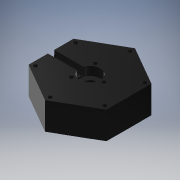
# Autodesk Inventor part: Spur Gear2
Saved by Autodesk Inventor 2017 (Build 210142000, 142)
## iProperties
Created: 2018-10-09
Part Number: Spur Gear2
Material: ABS Plastic
Document SubType Name: Modeling
Designer: Zach
Categories: <?xml version="1.0" encoding="UTF-16"?> <MemberInstance><Categories><FamilyTemplate><FamilyTemplateParameter ValueType="xs:double" Id="1" ObjectReferenceKey="da_z" ObjectType="kUserParameterObject"/><FamilyTemplateParameter ValueType="xs:double" Id="2" ObjectReferenceKey="da_b" ObjectType="kUserParameterObject"/><FamilyTemplateParameter ValueType="xs:double" Id="3" ObjectReferenceKey="da_beta" ObjectType="kUserParameterObject"/><FamilyTemplateParameter ValueType="xs:double" Id="4" ObjectReferenceKey="da_da" ObjectType="kUserParameterObject"/><FamilyTemplateParameter ValueType="xs:double" Id="5" ObjectReferenceKey="da_aw" ObjectType="kUserParameterObject"/><FamilyTemplateParameter ValueType="xs:string" Id="6" ObjectReferenceKey="EAIAABAAAACIAQAAAAAAAIAAAAAAAAAA" ObjectType="83910656" SubObjectId="SurfaceGeometry"/></FamilyTemplate><ParamToTemplateMap><ParamToTemplate CategoryParameter="//CategoryParameter[@InternalName='046C89C9-8512-4d59-83FE-43B91F4F132A']" TemplateParameter="1"/><ParamToTemplate CategoryParameter="//CategoryParameter[@InternalName='2552DF32-E462-4b46-AEBF-C6C7768E72AC']" TemplateParameter="2"/><ParamToTemplate CategoryParameter="//CategoryParameter[@InternalName='C9EE641D-15FC-4fae-A226-E94C4372FDD7']" TemplateParameter="3"/><ParamToTemplate><ParamToTemplate CategoryParameter="//CategoryParameter[@InternalName='00B6519A-459B-49c7-AD84-2E56D39A5744']" ConstantValue="0.000000"/></ParamToTemplate><ParamToTemplate><ParamToTemplate CategoryParameter="//CategoryParameter[@InternalName='04B31F0E-C7A6-4894-AA32-9629BEFACF47']" ConstantValue="1.000000"/></ParamToTemplate><ParamToTemplate><ParamToTemplate CategoryParameter="//CategoryParameter[@InternalName='43CBEC2E-7847-49e7-A936-2F7889FCB2D9']" ConstantValue="0.250000"/></ParamToTemplate><ParamToTemplate><ParamToTemplate CategoryParameter="//CategoryParameter[@InternalName='B1EFC894-105D-4ebd-86BF-FA20ED196853']" ConstantValue="0.350000"/></ParamToTemplate><ParamToTemplate><ParamToTemplate CategoryParameter="//CategoryParameter[@InternalName='51175063-3D10-4879-93E8-6246FE8B403D']" ConstantValue="2060000000.000000"/></ParamToTemplate><ParamToTemplate><ParamToTemplate CategoryParameter="//CategoryParameter[@InternalName='A3A52E27-4454-46a9-B0BD-C932399B70AF']" ConstantValue="0.300000"/></ParamToTemplate><ParamToTemplate><ParamToTemplate CategoryParameter="//CategoryParameter[@InternalName='91B76062-C214-41d9-B1B9-14D2AB99603D']" ConstantValue="0.200000"/></ParamToTemplate><ParamToTemplate><ParamToTemplate CategoryParameter="//CategoryParameter[@InternalName='374E806E-8B8A-4dda-A9AA-1039D6500AD2']" ConstantValue="5.000000"/></ParamToTemplate><ParamToTemplate><ParamToTemplate CategoryParameter="//CategoryParameter[@InternalName='2D373A89-B862-43d6-8D0B-0CBF12AB9F6C']" ConstantValue="0.392699"/></ParamToTemplate><ParamToTemplate CategoryParameter="//CategoryParameter[@InternalName='37777632-D6A2-4fac-9D53-DB8ACD95C989']" TemplateParameter="4"/><ParamToTemplate CategoryParameter="//CategoryParameter[@InternalName='FD1017F1-B727-4f7e-9707-0F86F1FF9423']" TemplateParameter="5"/><ParamToTemplate><ParamToTemplate CategoryParameter="//CategoryParameter[@InternalName='9E1B4470-B2D3-4ff1-B813-535BB4CDF51A']" ConstantValue="3520000.000000"/></ParamToTemplate><ParamToTemplate><ParamToTemplate CategoryParameter="//CategoryParameter[@InternalName='F8452263-BFF6-458c-9FB1-07C4B99E95CD']" ConstantValue="11400000.000000"/></ParamToTemplate><ParamToTemplate><ParamToTemplate CategoryParameter="//CategoryParameter[@InternalName='3E3BB259-FD49-497f-8171-6EBC954A3479']" ConstantValue="2.000000"/></ParamToTemplate><ParamToTemplate CategoryParameter="//CategoryParameter[@InternalName='27C3BAF2-7550-4e4b-AE2C-0DB134B7D9B7']" TemplateParameter="6"/></ParamToTemplateMap><Category DisplayName="Gear" InternalName="DC85795E-93AB-48d5-8EEE-5A27447B64BD" Mnemonic="Gear"><CategoryParameter DisplayName="z" InternalName="046C89C9-8512-4d59-83FE-43B91F4F132A" Mnemonic="z"/><CategoryParameter DisplayName="b" InternalName="2552DF32-E462-4b46-AEBF-C6C7768E72AC" Mnemonic="b"/><CategoryParameter DisplayName="||b|" InternalName="C9EE641D-15FC-4fae-A226-E94C4372FDD7" Mnemonic="beta"/><CategoryParameter DisplayName="x" InternalName="00B6519A-459B-49c7-AD84-2E56D39A5744" Mnemonic="x"/><CategoryParameter DisplayName="a*" InternalName="04B31F0E-C7A6-4894-AA32-9629BEFACF47" Mnemonic="a"/><CategoryParameter DisplayName="c*" InternalName="43CBEC2E-7847-49e7-A936-2F7889FCB2D9" Mnemonic="c"/><CategoryParameter DisplayName="r|.f|*" InternalName="B1EFC894-105D-4ebd-86BF-FA20ED196853" Mnemonic="rf"/><CategoryParameter DisplayName="E" InternalName="51175063-3D10-4879-93E8-6246FE8B403D" Mnemonic="E"/><CategoryParameter DisplayName="||m|" InternalName="A3A52E27-4454-46a9-B0BD-C932399B70AF" Mnemonic="mi"/><Category DisplayName="SpurGear" InternalName="26C5A22E-A91E-4dfd-A3B3-23CCAFAE1764" Mnemonic="SpurGear"><CategoryParameter DisplayName="m" InternalName="91B76062-C214-41d9-B1B9-14D2AB99603D" Mnemonic="m"/><CategoryParameter DisplayName="P" InternalName="374E806E-8B8A-4dda-A9AA-1039D6500AD2" Mnemonic="PP"/><CategoryParameter DisplayName="||a|" InternalName="2D373A89-B862-43d6-8D0B-0CBF12AB9F6C" Mnemonic="alpha"/><CategoryParameter DisplayName="d|.a|" InternalName="37777632-D6A2-4fac-9D53-DB8ACD95C989" Mnemonic="da"/><CategoryParameter DisplayName="a|.w|" InternalName="FD1017F1-B727-4f7e-9707-0F86F1FF9423" Mnemonic="aw"/><CategoryParameter DisplayName="||s||.Flim|" InternalName="9E1B4470-B2D3-4ff1-B813-535BB4CDF51A" Mnemonic="sFlim"/><CategoryParameter DisplayName="||s||.Hlim|" InternalName="F8452263-BFF6-458c-9FB1-07C4B99E95CD" Mnemonic="sHlim"/><CategoryParameter DisplayName="type" InternalName="3E3BB259-FD49-497f-8171-6EBC954A3479" Mnemonic="type"/><Category DisplayName="InternalSpurGear" InternalName="7CF704F6-14A9-42f8-93CE-E71DF57C2B55" Mnemonic="InternalSpurGear"><CategoryParameter DisplayName="PitchDiameter" InternalName="27C3BAF2-7550-4e4b-AE2C-0DB134B7D9B7" Mnemonic="IDS_PITCHDIAM"/></Category></Category></Category></Categories></MemberInstance>
Density: 1.06 g/cm^3
Appearance: Smooth - Black
CustomPartVersion: 0
Author: Zach
Autodesk Inventor part; units mm, degrees
ref_plane "YZ Plane" through (0, 0, 0) normal (1, 0, 0) x (0, 1, 0)
ref_plane "XZ Plane" through (0, 0, 0) normal (0, 1, 0) x (-1, 0, 0)
ref_plane "XY Plane" through (0, 0, 0) normal (0, 0, 1) x (1, 0, 0)
sketch "Sketch1" plane through (0, 0, 0) normal (0, 0, 1) x (1, 0, 0)
  circle A0 centre (0, 0) radius 52.25
  dimension "d0" = 104.5
  constraints: 1 centre point
  measures "d0" diameter of A0
extrude "Extrusion1" add sketch "Sketch1" along normal blind 10
ref_plane "Work Plane2" through (0, 0, 5) normal (0, 0, 1) x (1, 0, 0)
sketch "Sketch2" plane through (0, 0, 0) normal (0, 0, -1) x (-1, 0, 0)
  circle A0 centre (0, 0) radius 52.25 projected
  circle A1 centre (0, 0) radius 45
  dimension "d3" = 90
  constraints: 1 centre point, 1 coincident
  measures "d3" diameter of A1
surface extrude "Pitch Diameter" sketch "Sketch2" against normal through all shown no curves A1
ref_plane "Work Plane8" through (0, 0, 0) normal (0.9975641, 0.0697565, 0) x (0, 0, 1)
ref_plane "Work Plane9" through (0, 0, 0) normal (1, 0, 0) x (0, 1, 0)
spur gear teeth "Spur Gear" teeth 45 pitch diameter 90 tip diameter 86.2612 root diameter 95 face width 10 start plane through (0, 0, 0) normal (0, 0, -1) x (-1, 0, 0)
sketch "Sketch3" plane through (0, 0, 10) normal (0, 0, 1) x (1, 0, 0)
  arc A0 (2.2573, -43.0715) -> (3.7591, -42.9665) centre (0, 0) ccw projected
  arc A1 (0.829, -47.4928) -> (2.2573, -43.0715) centre (-19.4558, -38.4984) ccw projected
  arc A2 (-0.829, -47.4928) -> (0.829, -47.4928) centre (0, 0) ccw projected
  arc A3 (-2.2573, -43.0715) -> (-0.829, -47.4928) centre (19.4558, -38.4984) ccw projected
  arc A4 (-3.7591, -42.9665) -> (-2.2573, -43.0715) centre (0, 0) ccw projected
  arc A5 (-5.7888, -47.1459) -> (-3.7591, -42.9665) centre (-24.6244, -35.4161) ccw projected
  arc A6 (-7.4306, -46.9152) -> (-5.7888, -47.1459) centre (0, 0) ccw projected
  arc A7 (-8.2297, -42.3382) -> (-7.4306, -46.9152) centre (13.9085, -40.8315) ccw projected
  arc A8 (-9.7023, -42.0252) -> (-8.2297, -42.3382) centre (0, 0) ccw projected
  arc A9 (-12.2939, -45.8815) -> (-9.7023, -42.0252) centre (-29.3137, -31.6443) ccw projected
  arc A10 (-13.8877, -45.4245) -> (-12.2939, -45.8815) centre (0, 0) ccw projected
  arc A11 (-14.0419, -40.7808) -> (-13.8877, -45.4245) centre (8.0905, -42.3698) ccw projected
  arc A12 (-15.4566, -40.2659) -> (-14.0419, -40.7808) centre (0, 0) ccw projected
  arc A13 (-18.5597, -43.724) -> (-15.4566, -40.2659) centre (-33.4325, -27.2567) ccw projected
  arc A14 (-20.0744, -43.0496) -> (-18.5597, -43.724) centre (0, 0) ccw projected
  arc A15 (-19.5809, -38.4296) -> (-20.0744, -43.0496) centre (2.115, -43.0835) ccw projected
  arc A16 (-20.9101, -37.7229) -> (-19.5809, -38.4296) centre (0, 0) ccw projected
  arc A17 (-24.4643, -40.7154) -> (-20.9101, -37.7229) centre (-36.9005, -22.3385) ccw projected
  arc A18 (-25.8704, -39.8369) -> (-24.4643, -40.7154) centre (0, 0) ccw projected
  arc A19 (-24.7387, -35.3305) -> (-25.8704, -39.8369) centre (-3.9016, -42.9585) ccw projected
  arc A20 (-25.9566, -34.4456) -> (-24.7387, -35.3305) centre (0, 0) ccw projected
  arc A21 (-29.8927, -36.9144) -> (-25.9566, -34.4456) centre (-39.6503, -16.9856) ccw projected
  arc A22 (-31.1628, -35.8487) -> (-29.8927, -36.9144) centre (0, 0) ccw projected
  arc A23 (-29.415, -31.5437) -> (-31.1628, -35.8487) centre (-9.8423, -41.9975) ccw projected
  arc A24 (-30.4979, -30.4979) -> (-29.415, -31.5437) centre (0, 0) ccw projected
  arc A25 (-34.7393, -32.3949) -> (-30.4979, -30.4979) centre (-41.6284, -11.302) ccw projected
  arc A26 (-35.8487, -31.1628) -> (-34.7393, -32.3949) centre (0, 0) ccw projected
  arc A27 (-33.5188, -27.143) -> (-35.8487, -31.1628) centre (-15.5915, -40.219) ccw projected
  arc A28 (-34.4456, -25.9566) -> (-33.5188, -27.143) centre (0, 0) ccw projected
  arc A29 (-38.9097, -27.2449) -> (-34.4456, -25.9566) centre (-42.7962, -5.3985) ccw projected
  arc A30 (-39.8369, -25.8704) -> (-38.9097, -27.2449) centre (0, 0) ccw projected
  arc A31 (-36.9701, -22.2139) -> (-39.8369, -25.8704) centre (-21.0371, -37.6576) ccw projected
  arc A32 (-37.7229, -20.9101) -> (-36.9701, -22.2139) centre (0, 0) ccw projected
  arc A33 (-42.3228, -21.5645) -> (-37.7229, -20.9101) centre (-43.131, 0.6101) ccw projected
  arc A34 (-43.0496, -20.0744) -> (-42.3228, -21.5645) centre (0, 0) ccw projected
  arc A35 (-39.7019, -16.8525) -> (-43.0496, -20.0744) centre (-26.0733, -34.3634) ccw projected
  arc A36 (-40.2659, -15.4566) -> (-39.7019, -16.8525) centre (0, 0) ccw projected
  arc A37 (-44.9121, -15.4645) -> (-40.2659, -15.4566) centre (-42.6264, 6.6069) ccw projected
  arc A38 (-45.4245, -13.8877) -> (-44.9121, -15.4645) centre (0, 0) ccw projected
  arc A39 (-41.6609, -11.163) -> (-45.4245, -13.8877) centre (-30.602, -30.4002) ccw projected
  arc A40 (-42.0252, -9.7023) -> (-41.6609, -11.163) centre (0, 0) ccw projected
  arc A41 (-46.6273, -9.0634) -> (-42.0252, -9.7023) centre (-41.292, 12.475) ccw projected
  arc A42 (-46.9152, -7.4306) -> (-46.6273, -9.0634) centre (0, 0) ccw projected
  arc A43 (-42.8091, -5.2563) -> (-46.9152, -7.4306) centre (-34.5351, -25.8454) ccw projected
  arc A44 (-42.9665, -3.7591) -> (-42.8091, -5.2563) centre (0, 0) ccw projected
  arc A45 (-47.4349, -2.486) -> (-42.9665, -3.7591) centre (-39.154, 18.1004) ccw projected
  arc A46 (-47.4928, -0.829) -> (-47.4349, -2.486) centre (0, 0) ccw projected
  arc A47 (-43.124, 0.7527) -> (-47.4928, -0.829) centre (-37.796, -20.7875) ccw projected
  arc A48 (-43.0715, 2.2573) -> (-43.124, 0.7527) centre (0, 0) ccw projected
  arc A49 (-47.3192, 4.1399) -> (-43.0715, 2.2573) centre (-36.2539, 23.3734) ccw projected
  arc A50 (-47.1459, 5.7888) -> (-47.3192, 4.1399) centre (0, 0) ccw projected
  arc A51 (-42.5996, 6.7471) -> (-47.1459, 5.7888) centre (-40.3212, -15.325) ccw projected
  arc A52 (-42.3382, 8.2297) -> (-42.5996, 6.7471) centre (0, 0) ccw projected
  arc A53 (-46.2826, 10.6852) -> (-42.3382, 8.2297) centre (-32.6481, 28.1915) ccw projected
  arc A54 (-45.8815, 12.2939) -> (-46.2826, 10.6852) centre (0, 0) ccw projected
  arc A55 (-41.246, 12.6102) -> (-45.8815, 12.2939) centre (-42.0617, -9.5642) ccw projected
  arc A56 (-40.7808, 14.0419) -> (-41.246, 12.6102) centre (0, 0) ccw projected
  arc A57 (-44.3451, 17.0225) -> (-40.7808, 14.0419) centre (-28.4069, 32.4609) ccw projected
  arc A58 (-43.724, 18.5597) -> (-44.3451, 17.0225) centre (0, 0) ccw projected
  arc A59 (-39.0896, 18.2278) -> (-43.724, 18.5597) centre (-42.9834, -3.6173) ccw projected
  arc A60 (-38.4296, 19.5809) -> (-39.0896, 18.2278) centre (0, 0) ccw projected
  arc A61 (-41.5444, 23.0285) -> (-38.4296, 19.5809) centre (-23.6127, 36.0984) ccw projected
  arc A62 (-40.7154, 24.4643) -> (-41.5444, 23.0285) centre (0, 0) ccw projected
  arc A63 (-36.1724, 23.4906) -> (-40.7154, 24.4643) centre (-43.0685, 2.4) ccw projected
  arc A64 (-35.3305, 24.7387) -> (-36.1724, 23.4906) centre (0, 0) ccw projected
  arc A65 (-37.9352, 28.5862) -> (-35.3305, 24.7387) centre (-18.359, 39.0334) ccw projected
  arc A66 (-36.9144, 29.8927) -> (-37.9352, 28.5862) centre (0, 0) ccw projected
  arc A67 (-32.5511, 28.2962) -> (-36.9144, 29.8927) centre (-42.3154, 8.3706) ccw projected
  arc A68 (-31.5437, 29.415) -> (-32.5511, 28.2962) centre (0, 0) ccw projected
  arc A69 (-33.5876, 33.5876) -> (-31.5437, 29.415) centre (-12.748, 41.2086) ccw projected
  arc A70 (-32.3949, 34.7393) -> (-33.5876, 33.5876) centre (0, 0) ccw projected
  arc A71 (-28.2962, 32.5511) -> (-32.3949, 34.7393) centre (-40.7386, 14.1783) ccw projected
  arc A72 (-27.143, 33.5188) -> (-28.2962, 32.5511) centre (0, 0) ccw projected
  arc A73 (-28.5862, 37.9352) -> (-27.143, 33.5188) centre (-6.8888, 42.5817) ccw projected
  arc A74 (-27.2449, 38.9097) -> (-28.5862, 37.9352) centre (0, 0) ccw projected
  arc A75 (-23.4906, 36.1724) -> (-27.2449, 38.9097) centre (-38.3689, 19.7101) ccw projected
  arc A76 (-22.2139, 36.9701) -> (-23.4906, 36.1724) centre (0, 0) ccw projected
  arc A77 (-23.0285, 41.5444) -> (-22.2139, 36.9701) centre (-0.8955, 43.126) ccw projected
  arc A78 (-21.5645, 42.3228) -> (-23.0285, 41.5444) centre (0, 0) ccw projected
  arc A79 (-18.2278, 39.0896) -> (-21.5645, 42.3228) centre (-35.2524, 24.8582) ccw projected
  arc A80 (-16.8525, 39.7019) -> (-18.2278, 39.0896) centre (0, 0) ccw projected
  arc A81 (-17.0225, 44.3451) -> (-16.8525, 39.7019) centre (5.1152, 42.831) ccw projected
  arc A82 (-15.4645, 44.9121) -> (-17.0225, 44.3451) centre (0, 0) ccw projected
  arc A83 (-12.6102, 41.246) -> (-15.4645, 44.9121) centre (-31.4497, 29.5224) ccw projected
  arc A84 (-11.163, 41.6609) -> (-12.6102, 41.246) centre (0, 0) ccw projected
  arc A85 (-10.6852, 46.2826) -> (-11.163, 41.6609) centre (11.0263, 41.7022) ccw projected
  arc A86 (-9.0634, 46.6273) -> (-10.6852, 46.2826) centre (0, 0) ccw projected
  arc A87 (-6.7471, 42.5996) -> (-9.0634, 46.6273) centre (-27.0349, 33.6121) ccw projected
  arc A88 (-5.2563, 42.8091) -> (-6.7471, 42.5996) centre (0, 0) ccw projected
  arc A89 (-4.1399, 47.3192) -> (-5.2563, 42.8091) centre (16.7229, 39.7618) ccw projected
  arc A90 (-2.486, 47.4349) -> (-4.1399, 47.3192) centre (0, 0) ccw projected
  arc A91 (-0.7527, 43.124) -> (-2.486, 47.4349) centre (-22.0939, 37.0475) ccw projected
  arc A92 (0.7527, 43.124) -> (-0.7527, 43.124) centre (0, 0) ccw projected
  arc A93 (2.486, 47.4349) -> (0.7527, 43.124) centre (22.0939, 37.0475) ccw projected
  arc A94 (4.1399, 47.3192) -> (2.486, 47.4349) centre (0, 0) ccw projected
  arc A95 (5.2563, 42.8091) -> (4.1399, 47.3192) centre (-16.7229, 39.7618) ccw projected
  arc A96 (6.7471, 42.5996) -> (5.2563, 42.8091) centre (0, 0) ccw projected
  arc A97 (9.0634, 46.6273) -> (6.7471, 42.5996) centre (27.0349, 33.6121) ccw projected
  arc A98 (10.6852, 46.2826) -> (9.0634, 46.6273) centre (0, 0) ccw projected
  arc A99 (11.163, 41.6609) -> (10.6852, 46.2826) centre (-11.0263, 41.7022) ccw projected
  arc A100 (12.6102, 41.246) -> (11.163, 41.6609) centre (0, 0) ccw projected
  arc A101 (15.4645, 44.9121) -> (12.6102, 41.246) centre (31.4497, 29.5224) ccw projected
  arc A102 (17.0225, 44.3451) -> (15.4645, 44.9121) centre (0, 0) ccw projected
  arc A103 (16.8525, 39.7019) -> (17.0225, 44.3451) centre (-5.1152, 42.831) ccw projected
  arc A104 (18.2278, 39.0896) -> (16.8525, 39.7019) centre (0, 0) ccw projected
  arc A105 (21.5645, 42.3228) -> (18.2278, 39.0896) centre (35.2524, 24.8582) ccw projected
  arc A106 (23.0285, 41.5444) -> (21.5645, 42.3228) centre (0, 0) ccw projected
  arc A107 (22.2139, 36.9701) -> (23.0285, 41.5444) centre (0.8955, 43.126) ccw projected
  arc A108 (23.4906, 36.1724) -> (22.2139, 36.9701) centre (0, 0) ccw projected
  arc A109 (27.2449, 38.9097) -> (23.4906, 36.1724) centre (38.3689, 19.7101) ccw projected
  arc A110 (28.5862, 37.9352) -> (27.2449, 38.9097) centre (0, 0) ccw projected
  arc A111 (27.143, 33.5188) -> (28.5862, 37.9352) centre (6.8888, 42.5817) ccw projected
  arc A112 (28.2962, 32.5511) -> (27.143, 33.5188) centre (0, 0) ccw projected
  arc A113 (32.3949, 34.7393) -> (28.2962, 32.5511) centre (40.7386, 14.1783) ccw projected
  arc A114 (33.5876, 33.5876) -> (32.3949, 34.7393) centre (0, 0) ccw projected
  arc A115 (31.5437, 29.415) -> (33.5876, 33.5876) centre (12.748, 41.2086) ccw projected
  arc A116 (32.5511, 28.2962) -> (31.5437, 29.415) centre (0, 0) ccw projected
  arc A117 (36.9144, 29.8927) -> (32.5511, 28.2962) centre (42.3154, 8.3706) ccw projected
  arc A118 (37.9352, 28.5862) -> (36.9144, 29.8927) centre (0, 0) ccw projected
  arc A119 (35.3305, 24.7387) -> (37.9352, 28.5862) centre (18.359, 39.0334) ccw projected
  arc A120 (36.1724, 23.4906) -> (35.3305, 24.7387) centre (0, 0) ccw projected
  arc A121 (40.7154, 24.4643) -> (36.1724, 23.4906) centre (43.0685, 2.4) ccw projected
  arc A122 (41.5444, 23.0285) -> (40.7154, 24.4643) centre (0, 0) ccw projected
  arc A123 (38.4296, 19.5809) -> (41.5444, 23.0285) centre (23.6127, 36.0984) ccw projected
  arc A124 (39.0896, 18.2278) -> (38.4296, 19.5809) centre (0, 0) ccw projected
  arc A125 (43.724, 18.5597) -> (39.0896, 18.2278) centre (42.9834, -3.6173) ccw projected
  arc A126 (44.3451, 17.0225) -> (43.724, 18.5597) centre (0, 0) ccw projected
  arc A127 (40.7808, 14.0419) -> (44.3451, 17.0225) centre (28.4069, 32.4609) ccw projected
  arc A128 (41.246, 12.6102) -> (40.7808, 14.0419) centre (0, 0) ccw projected
  arc A129 (45.8815, 12.2939) -> (41.246, 12.6102) centre (42.0617, -9.5642) ccw projected
  arc A130 (46.2826, 10.6852) -> (45.8815, 12.2939) centre (0, 0) ccw projected
  arc A131 (42.3382, 8.2297) -> (46.2826, 10.6852) centre (32.6481, 28.1915) ccw projected
  arc A132 (42.5996, 6.7471) -> (42.3382, 8.2297) centre (0, 0) ccw projected
  arc A133 (47.1459, 5.7888) -> (42.5996, 6.7471) centre (40.3212, -15.325) ccw projected
  arc A134 (47.3192, 4.1399) -> (47.1459, 5.7888) centre (0, 0) ccw projected
  arc A135 (43.0715, 2.2573) -> (47.3192, 4.1399) centre (36.2539, 23.3734) ccw projected
  arc A136 (43.124, 0.7527) -> (43.0715, 2.2573) centre (0, 0) ccw projected
  arc A137 (47.4928, -0.829) -> (43.124, 0.7527) centre (37.796, -20.7875) ccw projected
  arc A138 (47.4349, -2.486) -> (47.4928, -0.829) centre (0, 0) ccw projected
  arc A139 (42.9665, -3.7591) -> (47.4349, -2.486) centre (39.154, 18.1004) ccw projected
  arc A140 (42.8091, -5.2563) -> (42.9665, -3.7591) centre (0, 0) ccw projected
  arc A141 (46.9152, -7.4306) -> (42.8091, -5.2563) centre (34.5351, -25.8454) ccw projected
  arc A142 (46.6273, -9.0634) -> (46.9152, -7.4306) centre (0, 0) ccw projected
  arc A143 (42.0252, -9.7023) -> (46.6273, -9.0634) centre (41.292, 12.475) ccw projected
  arc A144 (41.6609, -11.163) -> (42.0252, -9.7023) centre (0, 0) ccw projected
  arc A145 (45.4245, -13.8877) -> (41.6609, -11.163) centre (30.602, -30.4002) ccw projected
  arc A146 (44.9121, -15.4645) -> (45.4245, -13.8877) centre (0, 0) ccw projected
  arc A147 (40.2659, -15.4566) -> (44.9121, -15.4645) centre (42.6264, 6.6069) ccw projected
  arc A148 (39.7019, -16.8525) -> (40.2659, -15.4566) centre (0, 0) ccw projected
  arc A149 (43.0496, -20.0744) -> (39.7019, -16.8525) centre (26.0733, -34.3634) ccw projected
  arc A150 (42.3228, -21.5645) -> (43.0496, -20.0744) centre (0, 0) ccw projected
  arc A151 (37.7229, -20.9101) -> (42.3228, -21.5645) centre (43.131, 0.6101) ccw projected
  arc A152 (36.9701, -22.2139) -> (37.7229, -20.9101) centre (0, 0) ccw projected
  arc A153 (39.8369, -25.8704) -> (36.9701, -22.2139) centre (21.0371, -37.6576) ccw projected
  arc A154 (38.9097, -27.2449) -> (39.8369, -25.8704) centre (0, 0) ccw projected
  arc A155 (34.4456, -25.9566) -> (38.9097, -27.2449) centre (42.7962, -5.3985) ccw projected
  arc A156 (33.5188, -27.143) -> (34.4456, -25.9566) centre (0, 0) ccw projected
  arc A157 (35.8487, -31.1628) -> (33.5188, -27.143) centre (15.5915, -40.219) ccw projected
  arc A158 (34.7393, -32.3949) -> (35.8487, -31.1628) centre (0, 0) ccw projected
  arc A159 (30.4979, -30.4979) -> (34.7393, -32.3949) centre (41.6284, -11.302) ccw projected
  arc A160 (29.415, -31.5437) -> (30.4979, -30.4979) centre (0, 0) ccw projected
  arc A161 (31.1628, -35.8487) -> (29.415, -31.5437) centre (9.8423, -41.9975) ccw projected
  arc A162 (29.8927, -36.9144) -> (31.1628, -35.8487) centre (0, 0) ccw projected
  arc A163 (25.9566, -34.4456) -> (29.8927, -36.9144) centre (39.6503, -16.9856) ccw projected
  arc A164 (24.7387, -35.3305) -> (25.9566, -34.4456) centre (0, 0) ccw projected
  arc A165 (25.8704, -39.8369) -> (24.7387, -35.3305) centre (3.9016, -42.9585) ccw projected
  arc A166 (24.4643, -40.7154) -> (25.8704, -39.8369) centre (0, 0) ccw projected
  arc A167 (20.9101, -37.7229) -> (24.4643, -40.7154) centre (36.9005, -22.3385) ccw projected
  arc A168 (19.5809, -38.4296) -> (20.9101, -37.7229) centre (0, 0) ccw projected
  arc A169 (20.0744, -43.0496) -> (19.5809, -38.4296) centre (-2.115, -43.0835) ccw projected
  arc A170 (18.5597, -43.724) -> (20.0744, -43.0496) centre (0, 0) ccw projected
  arc A171 (15.4566, -40.2659) -> (18.5597, -43.724) centre (33.4325, -27.2567) ccw projected
  arc A172 (14.0419, -40.7808) -> (15.4566, -40.2659) centre (0, 0) ccw projected
  arc A173 (13.8877, -45.4245) -> (14.0419, -40.7808) centre (-8.0905, -42.3698) ccw projected
  arc A174 (12.2939, -45.8815) -> (13.8877, -45.4245) centre (0, 0) ccw projected
  arc A175 (9.7023, -42.0252) -> (12.2939, -45.8815) centre (29.3137, -31.6443) ccw projected
  arc A176 (8.2297, -42.3382) -> (9.7023, -42.0252) centre (0, 0) ccw projected
  arc A177 (7.4306, -46.9152) -> (8.2297, -42.3382) centre (-13.9085, -40.8315) ccw projected
  arc A178 (5.7888, -47.1459) -> (7.4306, -46.9152) centre (0, 0) ccw projected
  arc A179 (3.7591, -42.9665) -> (5.7888, -47.1459) centre (24.6244, -35.4161) ccw projected
  circle A180 centre (0, 0) radius 52.25 projected
extrude "Extrusion2" add sketch "Sketch3" along normal blind 10
sketch "Sketch4" plane through (0, 0, 20) normal (0, 0, 1) x (1, 0, 0)
  circle A0 centre (0, 0) radius 52.25 projected
  circle A1 centre (0, 0) radius 6.75
  circle A2 centre (30, 0) radius 3
  circle A3 centre (15, 25.9808) radius 3
  circle A4 centre (-15, 25.9808) radius 3
  circle A5 centre (-30, 0) radius 3
  circle A6 centre (-15, -25.9808) radius 3
  circle A7 centre (15, -25.9808) radius 3
  dimension "d55" = 13.5
  dimension "d56" = 6
  dimension "d57" = 30
  dimension "d60" = 360
  constraints: 7 centre point, 1 coincident, 1 horizontal alignment, 13 other
  measures "d55" diameter of A1
  measures "d56" diameter of A2
  measures "d57" distance of A2.centre point (0, 0)
extrude "Extrusion3" add sketch "Sketch4" along normal blind 15 contours A0 | A2 | A3 | A4 | A5 | A6 | A7
sketch "Sketch11" plane through (0, 0, 35) normal (0, 0, 1) x (1, 0, 0)
  circle A0 centre (0, 0) radius 52.25 projected
  circle A1 centre (0, 0) radius 57.5
  dimension "d96" = 115
  constraints: 1 centre point, 1 coincident
  measures "d96" diameter of A1
extrude "Extrusion9" add sketch "Sketch11" against normal blind 34.9
sketch "Sketch12" plane through (0, 0, 35) normal (0, 0, 1) x (1, 0, 0)
  circle A0 centre (0, 0) radius 6.75 projected
  line L0 (0, 57.5) -> (49.7965, 28.75)
  line L1 (49.7965, 28.75) -> (49.7965, -28.75)
  line L2 (49.7965, -28.75) -> (0, -57.5)
  line L3 (0, -57.5) -> (-49.7965, -28.75)
  line L4 (-49.7965, -28.75) -> (-49.7965, 28.75)
  line L5 (-49.7965, 28.75) -> (0, 57.5)
  circle A1 centre (0, 0) radius 57.5 projected
  constraints: 12 end point, 2 coincident, 2 vertical alignment, 14 other
extrude "Extrusion10" cut sketch "Sketch12" against normal through all contours A1 L0 | L5 A1 | A1 L1 | L4 A1 | A1 L2 | L3 A1
sketch "Sketch18" plane through (0, 0, 35) normal (0, 0, 1) x (1, 0, 0)
  circle A0 centre (17.5, 0) radius 2.5
  circle A1 centre (-8.75, 15.1554) radius 2.5
  circle A2 centre (-8.75, -15.1554) radius 2.5
  point P0 (0, 0)
  dimension "d133" = 5
  dimension "d134" = 17.5
  dimension "d137" = 360
  constraints: 3 centre point, 1 horizontal alignment, 7 other
  measures "d133" diameter of A0
  measures "d134" distance of point (0, 0) A0.centre
extrude "Extrusion15" cut sketch "Sketch18" against normal through all
sketch "Sketch20" plane through (0, 0, 35) normal (0, 0, 1) x (1, 0, 0)
  circle A0 centre (0, 51) radius 2.5
  circle A1 centre (-44.1673, 25.5) radius 2.5
  circle A2 centre (-44.1673, -25.5) radius 2.5
  circle A3 centre (0, -51) radius 2.5
  circle A4 centre (44.1673, -25.5) radius 2.5
  circle A5 centre (44.1673, 25.5) radius 2.5
  circle A6 centre (0, 0) radius 6.75 projected
  line L0 (0, -51) -> (0, 51)
  dimension "d155" = 5
  dimension "d159" = 360
  dimension "d198" = 102
  constraints: 6 centre point, 2 end point, 1 coincident, 1 vertical, 13 other
  measures "d155" diameter of A0
  measures "d198" distance of L0.start L0.end
extrude "Extrusion17" cut sketch "Sketch20" against normal through all contours A0 | A1 | A2 | A3 | A4 | A5
sketch "Sketch28" plane through (0, 0, 20) normal (0, 0, -1) x (-1, 0, 0)
  circle A0 centre (0, 0) radius 6.75 projected
  circle A1 centre (0, 0) radius 12
  dimension "d186" = 24
  constraints: 1 centre point, 1 coincident
  measures "d186" diameter of A1
extrude "Extrusion24" add sketch "Sketch28" along normal blind 20
sketch "Sketch29" plane through (0, 0, 35) normal (0, 0, 1) x (1, 0, 0)
  circle A0 centre (0, 0) radius 13
  dimension "d189" = 26
  constraints: 1 centre point, 1 coincident
  measures "d189" diameter of A0
extrude "Extrusion25" cut sketch "Sketch29" against normal blind 11.1
sketch "Sketch30" plane through (0, 0, 0) normal (1, 0, 0) x (0, 1, 0)
  circle A0 centre (0, 29.45) radius 4
  line L0 (-13, 35) -> (13, 35) projected
  point P0 (0, 0)
  point P1 (0, 35)
  dimension "d192" = 8
  dimension "d195" = 5.55
  constraints: 1 centre point, 1 midpoint, 1 vertical alignment
  measures "d192" diameter of A0
  measures "d195" distance from line of L0 A0.centre
extrude "Extrusion26" cut sketch "Sketch30" against normal through all
sketch "Sketch31" plane through (0, 0, 35) normal (0, 0, 1) x (1, 0, 0)
  line L0 (-49.7965, -4) -> (-49.7965, 4) projected
  line L1 (-49.7965, -4) -> (-3.0859, -4)
  line L2 (-3.0859, -4) -> (-3.0859, 4)
  line L3 (-3.0859, 4) -> (-49.7965, 4)
  line L4 (-49.7965, 4) -> (-49.7965, -4)
  point P0 (0, 0)
  constraints: 8 end point, 2 parallel, 1 horizontal, 1 perpendicular
extrude "Extrusion27" cut sketch "Sketch31" against normal blind 5.55
equation "\"d0\" = 1.1 * da_df"
equation "\"d1\" = da_b"
equation "\"d3\" = da_dw"
equation "\"da_df\" = 95"
equation "\"da_b\" = 10"
equation "\"da_dw\" = 90"
body "Solid1"
body "Srf1"
